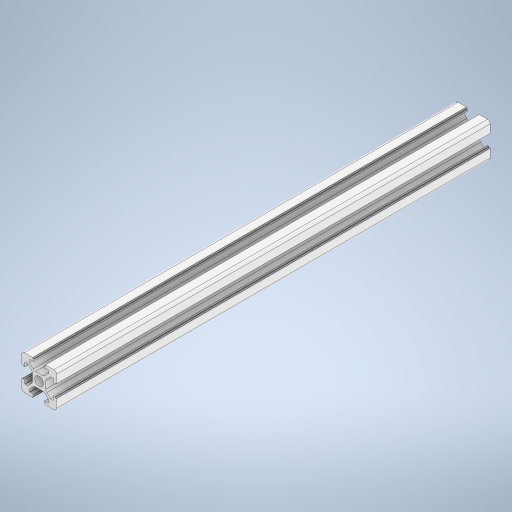
# Autodesk Inventor part: Extruded Alumnium 250mm
Saved by Autodesk Inventor 2024 (Build 280153000, 153)
## iProperties
Created: 2023-10-19
Part Number: Extruded Alumnium 250mm
Material: Aluminum 6063
Document SubType Name: Modeling
Designer: olson
Density: 2.68495 g/cm^3
Appearance: Default
Author: olson
Autodesk Inventor part; units mm, degrees
ref_plane "YZ Plane" through (0, 0, 0) normal (1, 0, 0) x (0, 1, 0)
ref_plane "XZ Plane" through (0, 0, 0) normal (0, 1, 0) x (-1, 0, 0)
ref_plane "XY Plane" through (0, 0, 0) normal (0, 0, 1) x (1, 0, 0)
sketch "Sketch1" plane through (0, 0, 0) normal (0, 0, 1) x (1, 0, 0)
  line L0 (-10, 10) -> (10, 10)
  line L1 (10, 10) -> (10, -10)
  line L2 (10, -10) -> (-10, -10)
  line L3 (-10, -10) -> (-10, 10)
  point P0 (0, 0)
  dimension "d3" = 20
  dimension "d4" = 20
  constraints: 8 end point, 2 parallel, 1 horizontal, 1 perpendicular
  measures "d3" distance of L1.end L2.end
  measures "d4" distance of L0.end L1.end
extrude "Extrusion1" add sketch "Sketch1" against normal blind 250
sketch "Sketch2" plane through (0, 0, 0) normal (0, 0, 1) x (1, 0, 0)
  circle A0 centre (0, 0) radius 2.5
  dimension "d7" = 5
  constraints: 1 centre point, 1 coincident
  measures "d7" diameter of A0
extrude "Extrusion2" cut sketch "Sketch2" against normal blind 250
sketch "Sketch3" plane through (0, 0, 0) normal (0, 0, 1) x (1, 0, 0)
  line L0 (-10, 10) -> (10, 10) projected
  line L1 (0, 3.9) -> (2.8393, 3.9)
  line L2 (0, 3.9) -> (-2.8393, 3.9)
  line L3 (0, 10) -> (-3.1, 10)
  line L4 (0, 10) -> (3.1, 10)
  line L5 (-3.1, 9.24) -> (-3.1, 8.2)
  line L6 (3.1, 9.24) -> (3.1, 8.2)
  line L7 (3.1, 8.2) -> (5.5, 8.2)
  line L8 (-3.1, 8.2) -> (-5.5, 8.2)
  line L9 (3.9, 3.9) -> (6.1627, 3.9) construction
  line L10 (-2.8393, 3.9) -> (-1.6373, 3.9) construction
  line L11 (-3.1, 10) -> (-3.6, 10)
  line L12 (-3.6, 10) -> (-3.6, 9.24)
  line L13 (-3.6, 9.24) -> (-3.1, 9.24)
  line L14 (3.1, 10) -> (3.6, 10)
  line L15 (3.6, 10) -> (3.6, 9.24)
  line L16 (3.6, 9.24) -> (3.1, 9.24)
  line L17 (-3.9, 3.9) -> (-3.15, 3.9) construction
  line L18 (-3.3697, 4.4303) -> (-2.8393, 3.9)
  line L19 (-3.3697, 4.4303) -> (-5.5, 6.5607)
  line L20 (-5.5, 6.5607) -> (-5.5, 8.2)
  line L21 (3.3697, 4.4303) -> (2.8393, 3.9)
  line L22 (3.3697, 4.4303) -> (5.5, 6.5607)
  line L23 (5.5, 6.5607) -> (5.5, 8.2)
  line L24 (-3.9, 0) -> (-3.9, 2.8393)
  line L25 (-3.9, 0) -> (-3.9, -2.8393)
  line L26 (-4.4303, -3.3697) -> (-6.5607, -5.5)
  line L27 (-4.4303, -3.3697) -> (-3.9, -2.8393)
  line L28 (-4.4303, 3.3697) -> (-3.9, 2.8393)
  line L29 (-4.4303, 3.3697) -> (-6.5607, 5.5)
  line L30 (-6.5607, 5.5) -> (-8.2, 5.5)
  line L31 (-8.2, 3.1) -> (-8.2, 5.5)
  line L32 (-9.24, 3.1) -> (-8.2, 3.1)
  line L33 (-9.24, 3.6) -> (-9.24, 3.1)
  line L34 (-10, 3.6) -> (-9.24, 3.6)
  line L35 (-10, 3.1) -> (-10, 3.6)
  line L36 (-10, 0) -> (-10, 3.1)
  line L37 (-10, 0) -> (-10, -3.1)
  line L38 (-10, -3.1) -> (-10, -3.6)
  line L39 (-10, -3.6) -> (-9.24, -3.6)
  line L40 (-9.24, -3.6) -> (-9.24, -3.1)
  line L41 (-9.24, -3.1) -> (-8.2, -3.1)
  line L42 (-8.2, -3.1) -> (-8.2, -5.5)
  line L43 (-6.5607, -5.5) -> (-8.2, -5.5)
  line L44 (0, -3.9) -> (-2.8393, -3.9)
  line L45 (0, -3.9) -> (2.8393, -3.9)
  line L46 (3.3697, -4.4303) -> (5.5, -6.5607)
  line L47 (3.3697, -4.4303) -> (2.8393, -3.9)
  line L48 (-3.3697, -4.4303) -> (-2.8393, -3.9)
  line L49 (-3.3697, -4.4303) -> (-5.5, -6.5607)
  line L50 (-5.5, -6.5607) -> (-5.5, -8.2)
  line L51 (-3.1, -8.2) -> (-5.5, -8.2)
  line L52 (-3.1, -9.24) -> (-3.1, -8.2)
  line L53 (-3.6, -9.24) -> (-3.1, -9.24)
  line L54 (-3.6, -10) -> (-3.6, -9.24)
  line L55 (-3.1, -10) -> (-3.6, -10)
  line L56 (0, -10) -> (-3.1, -10)
  line L57 (0, -10) -> (3.1, -10)
  line L58 (3.1, -10) -> (3.6, -10)
  line L59 (3.6, -10) -> (3.6, -9.24)
  line L60 (3.6, -9.24) -> (3.1, -9.24)
  line L61 (3.1, -9.24) -> (3.1, -8.2)
  line L62 (3.1, -8.2) -> (5.5, -8.2)
  line L63 (5.5, -6.5607) -> (5.5, -8.2)
  line L64 (3.9, 0) -> (3.9, -2.8393)
  line L65 (3.9, 0) -> (3.9, 2.8393)
  line L66 (4.4303, 3.3697) -> (6.5607, 5.5)
  line L67 (4.4303, 3.3697) -> (3.9, 2.8393)
  line L68 (4.4303, -3.3697) -> (3.9, -2.8393)
  line L69 (4.4303, -3.3697) -> (6.5607, -5.5)
  line L70 (6.5607, -5.5) -> (8.2, -5.5)
  line L71 (8.2, -3.1) -> (8.2, -5.5)
  line L72 (9.24, -3.1) -> (8.2, -3.1)
  line L73 (9.24, -3.6) -> (9.24, -3.1)
  line L74 (10, -3.6) -> (9.24, -3.6)
  line L75 (10, -3.1) -> (10, -3.6)
  line L76 (10, 0) -> (10, -3.1)
  line L77 (10, 0) -> (10, 3.1)
  line L78 (10, 3.1) -> (10, 3.6)
  line L79 (10, 3.6) -> (9.24, 3.6)
  line L80 (9.24, 3.6) -> (9.24, 3.1)
  line L81 (9.24, 3.1) -> (8.2, 3.1)
  line L82 (8.2, 3.1) -> (8.2, 5.5)
  line L83 (6.5607, 5.5) -> (8.2, 5.5)
  point P0 (0, 0)
  dimension "d11" = 3.9
  dimension "d12" = 3.9
  dimension "d13" = 3.1
  dimension "d14" = 3.1
  dimension "d15" = 1.8
  dimension "d16" = 1.8
  dimension "d17" = 2.4
  dimension "d18" = 2.4
  dimension "d30" = 0.5
  dimension "d31" = 0.76
  dimension "d32" = 0.5
  dimension "d33" = 0.76
  dimension "d40" = 360
  constraints: 166 end point, 16 point on line, 6 horizontal, 4 perpendicular, 2 vertical, 1 midpoint, 1 parallel, 161 other
  measures "d11" distance of L1.start L9.start
  measures "d12" distance of L1.start L17.start
  measures "d13" distance of L3.start L3.end
  measures "d14" distance of L3.start L4.end
  measures "d15" distance of L3.end L5.end
  measures "d16" distance of L4.end L6.end
  measures "d17" distance of L6.end L7.end
  measures "d18" distance of L5.end L8.end
  measures "d30" distance of L3.end L11.end
  measures "d31" distance of L11.end L12.end
  measures "d32" distance of L4.end L14.end
  measures "d33" distance of L14.end L15.end
extrude "Extrusion3" cut sketch "Sketch3" against normal blind 250
fillet "Fillet2" radius 2 8 edges at (-2.8393, 3.9, -125) (2.8393, 3.9, -125) (3.9, 2.8393, -125) (3.9, -2.8393, -125) (2.8393, -3.9, -125) (-2.8393, -3.9, -125) (-3.9, -2.8393, -125) (-3.9, 2.8393, -125)
fillet "Fillet4" radius 1.5 4 edges at (10, 10, -125) (10, -10, -125) (-10, -10, -125) (-10, 10, -125)
fillet "Fillet5" radius 0.1 40 edges at (8.2, -5.5, -125) (8.2, -3.1, -125) (9.24, -3.1, -125) (9.24, -3.6, -125) (10, -3.6, -125) (10, 3.6, -125) (9.24, 3.6, -125) (9.24, 3.1, -125) (8.2, 3.1, -125) (8.2, 5.5, -125) (3.6, 10, -125) (3.6, 9.24, -125) (3.1, 9.24, -125) (3.1, 8.2, -125) (5.5, 8.2, -125) (-5.5, 8.2, -125) (-3.1, 8.2, -125) (-3.1, 9.24, -125) (-3.6, 9.24, -125) (-3.6, 10, -125) (-8.2, 5.5, -125) (-8.2, 3.1, -125) (-9.24, 3.1, -125) (-9.24, 3.6, -125) (-10, 3.6, -125) (-8.2, -3.1, -125) (-8.2, -5.5, -125) (-9.24, -3.1, -125) (-9.24, -3.6, -125) (-10, -3.6, -125) (-3.1, -8.2, -125) (-5.5, -8.2, -125) (-3.1, -9.24, -125) (-3.6, -9.24, -125) (-3.6, -10, -125) (5.5, -8.2, -125) (3.1, -8.2, -125) (3.1, -9.24, -125) (3.6, -9.24, -125) (3.6, -10, -125)
body "Solid1"
